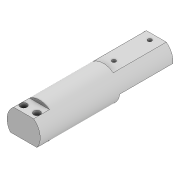
# Autodesk Inventor part: link2
Saved by Autodesk Inventor 2022 (Build 260153000, 153)
## iProperties
Created: 2022-02-15
Part Number: link2
Material: Generic
Document SubType Name: Modeling
Designer: New-Computer
Density: 1 g/cm^3
Appearance: Default
Mass: 2187.16 g
Surface Area: 1296.73 cm^2
Volume: 2187.16 cm^3
Author: New-Computer
Autodesk Inventor part; units mm, degrees
ref_plane "YZ Plane" through (0, 0, 0) normal (1, 0, 0) x (0, 1, 0)
ref_plane "XZ Plane" through (0, 0, 0) normal (0, 1, 0) x (-1, 0, 0)
ref_plane "XY Plane" through (0, 0, 0) normal (0, 0, 1) x (1, 0, 0)
sketch "Sketch1" plane through (0, 0, 0) normal (0, 0, 1) x (1, 0, 0)
  circle A0 centre (0, 0) radius 12.5
  dimension "d0" = 25
  constraints: 1 centre point, 1 coincident
  measures "d0" diameter of A0
extrude "Extrusion1" add sketch "Sketch1" along normal blind 60
sketch "Sketch14" plane through (0, 0, 0) normal (0, 0, -1) x (-1, 0, 0)
  line L0 (0, 0) -> (0, 1.5)
  circle A0 centre (0, 0) radius 12.5 projected
  line L1 (0, 1.5) -> (-12.4097, 1.5)
  line L2 (0, 0) -> (-1.8933, 0)
  line L3 (0, 1.5) -> (12.4097, 1.5)
  line L4 (0, -1.5) -> (-12.4097, -1.5)
  line L5 (0, -1.5) -> (12.4097, -1.5)
  dimension "d71" = 1.5
  constraints: 12 end point, 4 symmetric about line, 2 horizontal, 1 vertical, 2 other
  measures "d71" distance of L0.start L0.end
extrude "Extrusion10" add sketch "Sketch14" along normal blind 40 contours A0 L5 L4 L1 L3
sketch "Sketch16" plane through (0, 0, 60) normal (0, 0, 1) x (1, 0, 0)
  arc A0 (-12.4097, -1.5) -> (12.4097, -1.5) centre (0, 0) ccw projected
  line L0 (-10, -7.5) -> (10, -7.5)
  line L1 (12.4097, -1.5) -> (-12.4097, -1.5) projected
  dimension "d83" = 20
  constraints: 2 end point, 2 point on circle, 1 parallel
  measures "d83" distance of L0.start L0.end
extrude "Extrusion12" cut sketch "Sketch16" against normal blind 10 contours L0 A0
sketch "Sketch17" plane through (0, 0, 0) normal (0, 0, -1) x (-1, 0, 0)
  line L0 (-12.4097, 1.5) -> (12.4097, 1.5) projected
  arc A0 (12.4097, 1.5) -> (-12.4097, 1.5) centre (0, 0) ccw projected
extrude "Extrusion13" add sketch "Sketch17" along normal up to surface (40 mm away)
sketch "Sketch15" plane through (-12.4097, 1.5, 0) normal (0, 1, 0) x (1, 0, 0)
  line L0 (0, 0) -> (0, 40) projected
  line L1 (0, 40) -> (24.8193, 40) projected
  circle A0 centre (12.4097, 35) radius 1.5
  circle A1 centre (12.4097, 8) radius 1.5
  point P0 (12.4097, 0)
  dimension "d79" = 3
  dimension "d80" = 5
  dimension "d81" = 3
  dimension "d82" = 27
  constraints: 2 centre point
  measures "d79" diameter of A0
  measures "d80" distance from line of L1 A0.centre
  measures "d81" diameter of A1
  measures "d82" distance of A1.centre A0.centre
extrude "Extrusion11" cut sketch "Sketch15" along normal mid plane 22
sketch "Sketch18" plane through (-10, -7.5, 60) normal (0, -1, 0) x (1, 0, 0)
  arc A0 (6.5, -7) -> (3.5, -7) centre (5, -5) ccw projected
  arc A1 (16.5, -7) -> (13.5, -7) centre (15, -5) ccw projected
  circle A2 centre (5, -5) radius 2.5
  circle A3 centre (15, -5) radius 2.5
  point P0 (10, -60)
  point P1 (13.5, -7)
  point P2 (16.5, -7)
  point P3 (3.5, -7)
  point P4 (6.5, -7)
  constraints: 2 centre point, 2 coincident, 2 concentric
extrude "Extrusion14" cut sketch "Sketch18" against normal blind 22
sketch "Sketch19" plane through (0, 0, -40) normal (0, 0, -1) x (-1, 0, 0)
  arc A0 (12.4097, -1.5) -> (-12.4097, -1.5) centre (0, 0) ccw projected
  line L0 (7.5, 10) -> (-7.5, 10)
  dimension "d90" = 15
  constraints: 2 end point, 2 point on circle, 1 horizontal
  measures "d90" distance of L0.start L0.end
extrude "Extrusion15" cut sketch "Sketch19" against normal blind 40
sketch "Sketch20" plane through (0, 0, 60) normal (0, 0, 1) x (1, 0, 0)
  arc A0 (10, -7.5) -> (-10, -7.5) centre (0, 0) ccw projected
  line L0 (-7.5, 10) -> (7.5, 10)
  dimension "d93" = 15
  constraints: 2 end point, 2 point on circle, 1 horizontal
  measures "d93" distance of L0.start L0.end
extrude "Extrusion16" cut sketch "Sketch20" against normal blind 12
body "Solid1"
